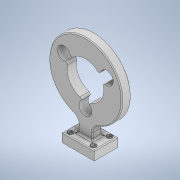
# Autodesk Inventor part: держалка_для_мозговорота
Saved by Autodesk Inventor 2021 (Build 250183000, 183)
## iProperties
Created: 2022-11-11
Part Number: держалка_для_мозговорота
Material: Типовые
Document SubType Name: Modeling
Designer: zmoze
Density: 1 g/cm^3
Appearance: По умолчанию
Author: zmoze
Autodesk Inventor part; units mm, degrees
ref_plane "YZ Plane" through (0, 0, 0) normal (1, 0, 0) x (0, 1, 0)
sketch "Эскиз1" plane through (0, 0, 0) normal (0, 0, 1) x (1, 0, 0)
  circle A0 centre (0, 59.2906) radius 20.05
  circle A1 centre (0, 32.1906) radius 7.05
  line L0 (0, 119.1487) -> (0, -19.8581) projected
  circle A2 centre (0, 59.2906) radius 40
  line L1 (-7.5, 0) -> (7.5, 0)
  line L2 (-7.5, 20) -> (-7.5, 0)
  line L3 (7.5, 0) -> (7.5, 20)
  line L4 (-56, 0) -> (56, 0) projected
  line L5 (0, 59.2906) -> (-2.711, 38.6985)
  line L6 (0, 59.2906) -> (2.711, 38.6985)
  line L7 (0, 59.2906) -> (16.4778, 71.9344)
  line L8 (0, 59.2906) -> (19.1888, 67.2388)
  circle A3 centre (23.4693, 72.8406) radius 7.05
  line L9 (0, 59.2906) -> (-19.1888, 67.2388)
  line L10 (0, 59.2906) -> (-16.4778, 71.9344)
  circle A4 centre (-23.4693, 72.8406) radius 7.05
  point P0 (0, 0)
  point P1 (0, 39.2406)
  point P2 (-2.6171, 39.4121)
  point P3 (-18.5238, 66.9634)
  point P4 (-15.9067, 71.4963)
  point P5 (15.9067, 71.4963)
  point P6 (18.5238, 66.9634)
  point P7 (2.6171, 39.4121)
  dimension "d0" = 40.1
  dimension "d5" = 14.1
  dimension "d10" = 80
  dimension "d11" = 15
  dimension "d12" = 20
  dimension "d17" = 15
  dimension "d20" = 360
  constraints: 18 end point, 8 point on circle, 5 centre point, 2 point on line, 1 coincident, 1 equal length, 1 horizontal, 1 midpoint, 1 parallel, 1 tangent, 1 vertical, 22 other
  measures "d0" diameter of A0
  measures "d5" diameter of A1
  measures "d10" diameter of A2
  measures "d11" distance between parallel lines of L3 L2
  measures "d12" distance of L1.end L3.end
  measures "d17" angle of L6 L5
extrude "Выдавливание1" add sketch "Эскиз1" along normal blind 10 contours A0 L8 A3 L7 L0 A2 A1 L6 | A0 L10 A4 L9 L5 A1 L0 A2 | A2 L3 L1 L0 | L0 L1 L2 A2
fillet "Сопряжение1" radius 2 12 edges at (-16.4778, 71.9344, 5) (-15.9067, 71.4963, 5) (-19.1888, 67.2388, 5) (-18.5238, 66.9634, 5) (16.4778, 71.9344, 5) (15.9067, 71.4963, 5) (19.1888, 67.2388, 5) (18.5238, 66.9634, 5) (-2.6171, 39.4121, 5) (-2.711, 38.6985, 5) (2.6171, 39.4121, 5) (2.711, 38.6985, 5)
fillet "Сопряжение2" radius 10 2 edges at (7.5, 20, 5) (-7.5, 20, 5)
sketch "Эскиз2" plane through (-7.5, 0, 0) normal (0, -1, 0) x (1, 0, 0)
  line L0 (-10, 18) -> (25, 18)
  line L1 (25, 18) -> (25, -8)
  line L2 (25, -8) -> (-10, -8)
  line L3 (-10, -8) -> (-10, 18)
  line L4 (7.5, 0) -> (7.5, 10) construction
  line L5 (-6.001, 10) -> (21.001, 10) construction
  line L6 (7.5, 23.2) -> (7.5, -13.2) construction
  line L7 (0, 0) -> (15, 0) construction
  line L8 (15, 0) -> (15, 10) construction
  point P0 (7.5, -8)
  dimension "d24" = 8
  dimension "d25" = 8
  dimension "d26" = 10
  constraints: 10 end point, 2 midpoint, 2 parallel, 1 horizontal, 1 perpendicular, 1 point on line
  measures "d24" distance between parallel lines of L2 L7
  measures "d25" distance between parallel lines of L0 L5
  measures "d26" distance between parallel lines of L8 L1
extrude "Выдавливание2" add sketch "Эскиз2" along normal blind 5 and the other way blind 5
sketch "Эскиз3" plane through (-7.5, 5, 0) normal (0, 1, 0) x (1, 0, 0)
  circle A0 centre (-5, 3.75) radius 1.5
  line L0 (-4.134, 5.25) -> (-3.2679, 3.75)
  line L1 (-3.2679, 3.75) -> (-4.134, 2.25)
  line L2 (-4.134, 2.25) -> (-5.866, 2.25)
  line L3 (-5.866, 2.25) -> (-6.7321, 3.75)
  line L4 (-6.7321, 3.75) -> (-5.866, 5.25)
  line L5 (-5.866, 5.25) -> (-4.134, 5.25)
  line L6 (-1.8246, 3.75) -> (-3.4123, 6.5)
  line L7 (-3.4123, 6.5) -> (-6.5877, 6.5)
  line L8 (-6.5877, 6.5) -> (-8.1754, 3.75)
  line L9 (-8.1754, 3.75) -> (-6.5877, 1)
  line L10 (-6.5877, 1) -> (-3.4123, 1)
  line L11 (-3.4123, 1) -> (-1.8246, 3.75)
  circle A1 centre (-5, -13.75) radius 1.5
  line L12 (-4.134, -12.25) -> (-3.2679, -13.75)
  line L13 (-3.2679, -13.75) -> (-4.134, -15.25)
  line L14 (-4.134, -15.25) -> (-5.866, -15.25)
  line L15 (-5.866, -15.25) -> (-6.7321, -13.75)
  line L16 (-6.7321, -13.75) -> (-5.866, -12.25)
  line L17 (-5.866, -12.25) -> (-4.134, -12.25)
  line L18 (-1.8246, -13.75) -> (-3.4123, -11)
  line L19 (-3.4123, -11) -> (-6.5877, -11)
  line L20 (-6.5877, -11) -> (-8.1754, -13.75)
  line L21 (-8.1754, -13.75) -> (-6.5877, -16.5)
  line L22 (-6.5877, -16.5) -> (-3.4123, -16.5)
  line L23 (-3.4123, -16.5) -> (-1.8246, -13.75)
  circle A2 centre (20, 3.75) radius 1.5
  line L24 (20.866, 5.25) -> (21.7321, 3.75)
  line L25 (21.7321, 3.75) -> (20.866, 2.25)
  line L26 (20.866, 2.25) -> (19.134, 2.25)
  line L27 (19.134, 2.25) -> (18.2679, 3.75)
  line L28 (18.2679, 3.75) -> (19.134, 5.25)
  line L29 (19.134, 5.25) -> (20.866, 5.25)
  line L30 (23.1754, 3.75) -> (21.5877, 6.5)
  line L31 (21.5877, 6.5) -> (18.4123, 6.5)
  line L32 (18.4123, 6.5) -> (16.8246, 3.75)
  line L33 (16.8246, 3.75) -> (18.4123, 1)
  line L34 (18.4123, 1) -> (21.5877, 1)
  line L35 (21.5877, 1) -> (23.1754, 3.75)
  circle A3 centre (20, -13.75) radius 1.5
  line L36 (20.866, -12.25) -> (21.7321, -13.75)
  line L37 (21.7321, -13.75) -> (20.866, -15.25)
  line L38 (20.866, -15.25) -> (19.134, -15.25)
  line L39 (19.134, -15.25) -> (18.2679, -13.75)
  line L40 (18.2679, -13.75) -> (19.134, -12.25)
  line L41 (19.134, -12.25) -> (20.866, -12.25)
  line L42 (23.1754, -13.75) -> (21.5877, -11)
  line L43 (21.5877, -11) -> (18.4123, -11)
  line L44 (18.4123, -11) -> (16.8246, -13.75)
  line L45 (16.8246, -13.75) -> (18.4123, -16.5)
  line L46 (18.4123, -16.5) -> (21.5877, -16.5)
  line L47 (21.5877, -16.5) -> (23.1754, -13.75)
  line L48 (-5, 3.75) -> (20, 3.75) construction
  line L49 (20, 3.75) -> (20, -13.75) construction
  line L50 (20, -13.75) -> (-5, -13.75) construction
  line L51 (-5, -13.75) -> (-5, 3.75) construction
  line L52 (25, 8) -> (-10, 8) construction
  line L53 (-10, 8) -> (-10, -18) construction
  line L54 (25, -18) -> (25, 8) construction
  line L55 (-10, -18) -> (25, -18) construction
  point P0 (-5, 5.25)
  point P1 (-5, -12.25)
  point P2 (20, 5.25)
  point P3 (20, -12.25)
  dimension "d32" = 3
  dimension "d34" = 3
  dimension "d36" = 3
  dimension "d38" = 3
  dimension "d33" = 5.5
  dimension "d35" = 5.5
  dimension "d37" = 5.5
  dimension "d39" = 5.5
  dimension "d40" = 1.5
  dimension "d41" = 5
  dimension "d42" = 5
  dimension "d43" = 1.5
  constraints: 104 end point, 6 horizontal, 5 coincident, 4 midpoint, 4 vertical alignment, 2 vertical, 80 other
  measures "d33" distance between parallel lines of L10 L7
  measures "d35" distance between parallel lines of L22 L19
  measures "d37" distance between parallel lines of L34 L31
  measures "d39" distance between parallel lines of L46 L43
  measures "d40" distance between parallel lines of L52 L7
  measures "d41" distance from line of L53 point (-5, 3.75)
  measures "d42" distance from line of point (20, 3.75) L54
  measures "d43" distance between parallel lines of L55 L46
extrude "Выдавливание3" cut sketch "Эскиз3" against normal blind 2.5 contours A0 | A0 L0 L1 | A0 L5 L0 | L1 L2 A0 | A0 L4 L5 | L2 L3 A0 | A0 L3 L4 | L11 L10 L9 L8 L7 L6 | A1 | A1 L12 L13 | A1 L17 L12 | L13 L14 A1 | A1 L16 L17 | L14 L15 A1 | A1 L15 L16 | L23 L22 L21 L20 L19 L18 | A2 | A2 L24 L25 | A2 L29 L24 | L25 L26 A2 | A2 L28 L29 | L26 L27 A2 | A2 L27 L28 | L35 L34 L33 L32 L31 L30 | A3 | A3 L36 L37 | A3 L41 L36 | L37 L38 A3 | A3 L40 L41 | L38 L39 A3 | A3 L39 L40 | L47 L46 L45 L44 L43 L42
sketch "Эскиз4" plane through (-7.5, 5, 0) normal (0, 1, 0) x (1, 0, 0)
  line L0 (-6.5877, 6.5) -> (-3.4123, 6.5) projected
  line L1 (-8.1754, 3.75) -> (-6.5877, 6.5) projected
  line L2 (-6.5877, 1) -> (-8.1754, 3.75) projected
  line L3 (-3.4123, 1) -> (-6.5877, 1) projected
  line L4 (-1.8246, 3.75) -> (-3.4123, 1) projected
  line L5 (-3.4123, 6.5) -> (-1.8246, 3.75) projected
  line L6 (18.4123, 6.5) -> (21.5877, 6.5) projected
  line L7 (16.8246, 3.75) -> (18.4123, 6.5) projected
  line L8 (18.4123, 1) -> (16.8246, 3.75) projected
  line L9 (21.5877, 1) -> (18.4123, 1) projected
  line L10 (23.1754, 3.75) -> (21.5877, 1) projected
  line L11 (21.5877, 6.5) -> (23.1754, 3.75) projected
  line L12 (18.4123, -11) -> (21.5877, -11) projected
  line L13 (16.8246, -13.75) -> (18.4123, -11) projected
  line L14 (18.4123, -16.5) -> (16.8246, -13.75) projected
  line L15 (21.5877, -16.5) -> (18.4123, -16.5) projected
  line L16 (23.1754, -13.75) -> (21.5877, -16.5) projected
  line L17 (21.5877, -11) -> (23.1754, -13.75) projected
  line L18 (-6.5877, -11) -> (-3.4123, -11) projected
  line L19 (-8.1754, -13.75) -> (-6.5877, -11) projected
  line L20 (-6.5877, -16.5) -> (-8.1754, -13.75) projected
  line L21 (-3.4123, -16.5) -> (-6.5877, -16.5) projected
  line L22 (-1.8246, -13.75) -> (-3.4123, -16.5) projected
  line L23 (-3.4123, -11) -> (-1.8246, -13.75) projected
  circle A0 centre (-5, 3.75) radius 2.75
  circle A1 centre (20, 3.75) radius 2.75
  circle A2 centre (20, -13.75) radius 2.75
  circle A3 centre (-5, -13.75) radius 2.75
  circle A4 centre (-5, 3.75) radius 1.5
  circle A5 centre (20, 3.75) radius 1.5
  circle A6 centre (20, -13.75) radius 1.5
  circle A7 centre (-5, -13.75) radius 1.5
  point P0 (7.5, 0)
  dimension "d46" = 3
  constraints: 12 tangent, 8 centre point, 4 coincident, 3 equal radius
  measures "d46" diameter of A4
extrude "Выдавливание4" cut sketch "Эскиз4" against normal up to surface (10 mm away) contours A4 | A5 | A6 | A7
fillet "Сопряжение3" radius 2 4 edges at (0, 5, 10) (-7.5, 5, 5) (7.5, 5, 5) (0, 5, 0)
fillet "Сопряжение4" radius 1 18 edges at (-9.2842, 18.154, 10) (-7.5, 9.7265, 10) (-8.0858, 5.5858, 10.5858) (9.2842, 18.154, 10) (7.5, 9.7265, 10) (8.0858, 5.5858, 10.5858) (0, 99.2906, 10) (-9.2842, 18.154, 0) (-7.5, 9.7265, 0) (-8.0858, 5.5858, -0.5858) (9.2842, 18.154, 0) (7.5, 9.7265, 0) (8.0858, 5.5858, -0.5858) (0, 99.2906, 0) (-17.5, 5, 5) (0, 5, -8) (17.5, 5, 5) (0, 5, 18)
ref_plane "РабПлоскость1" through (17.5, -5, 5) normal (0, 0, -1) x (-1, 0, 0)
ref_plane "РабПлоскость2" through (0, -5, -8) normal (-1, 0, 0) x (0, 0, 1)
